Autodesk Inventor part; units mm, degrees
(part 3 of 3)
sketch "Sketch6" plane through (0, 0, 1.2) normal (0, 0, -1) x (-1, 0, 0)
  line L0 (5.715, -18.5) -> (4.445, -18.5) construction
  line L1 (4.445, -18.5) -> (4.445, -20.9) construction
  line L2 (4.445, -20.9) -> (5.715, -20.9) projected
  line L3 (5.715, -20.9) -> (5.715, -18.5) construction
  line L4 (3.175, -18.5) -> (1.905, -18.5) construction
  line L5 (1.905, -18.5) -> (1.905, -20.9) construction
  line L6 (1.905, -20.9) -> (3.175, -20.9) projected
  line L7 (3.175, -20.9) -> (3.175, -18.5) construction
  line L8 (0.635, -18.5) -> (-0.635, -18.5) construction
  line L9 (-0.635, -18.5) -> (-0.635, -20.9) construction
  line L10 (-0.635, -20.9) -> (0.635, -20.9) projected
  line L11 (0.635, -20.9) -> (0.635, -18.5) construction
  line L12 (-1.905, -18.5) -> (-3.175, -18.5) construction
  line L13 (-3.175, -18.5) -> (-3.175, -20.9) construction
  line L14 (-3.175, -20.9) -> (-1.905, -20.9) projected
  line L15 (-1.905, -20.9) -> (-1.905, -18.5) construction
  line L16 (-4.445, -18.5) -> (-5.715, -18.5) construction
  line L17 (-5.715, -18.5) -> (-5.715, -20.9) construction
  line L18 (-5.715, -20.9) -> (-4.445, -20.9) projected
  line L19 (-4.445, -20.9) -> (-4.445, -18.5) construction
  line L20 (-20.14, 20.9) -> (-21.39, 20.9) construction
  line L21 (-21.39, 20.9) -> (-21.39, 18.5) construction
  line L22 (-21.39, 18.5) -> (-20.14, 18.5) construction
  line L23 (-20.14, 18.5) -> (-20.14, 20.9) construction
  line L24 (-17.6, 20.9) -> (-18.85, 20.9) construction
  line L25 (-18.85, 20.9) -> (-18.85, 18.5) construction
  line L26 (-18.85, 18.5) -> (-17.6, 18.5) construction
  line L27 (-17.6, 18.5) -> (-17.6, 20.9) construction
  line L28 (21.39, 20.9) -> (20.14, 20.9) construction
  line L29 (20.14, 20.9) -> (20.14, 18.5) construction
  line L30 (20.14, 18.5) -> (21.39, 18.5) construction
  line L31 (21.39, 18.5) -> (21.39, 20.9) construction
  line L32 (18.85, 20.9) -> (17.6, 20.9) construction
  line L33 (17.6, 20.9) -> (17.6, 18.5) construction
  line L34 (17.6, 18.5) -> (18.85, 18.5) construction
  line L35 (18.85, 18.5) -> (18.85, 20.9) construction
  line L36 (5.715, -20.9) -> (4.445, -20.9) projected
  line L37 (4.445, -20.9) -> (4.445, -18.5) construction
  line L38 (5.715, -20.9) -> (4.445, -20.9)
  line L39 (4.445, -20.9) -> (4.445, -20.6)
  line L40 (4.445, -20.6) -> (5.715, -20.6)
  line L41 (5.715, -20.6) -> (5.715, -20.9)
  line L42 (3.175, -18.5) -> (3.175, -20.9) construction
  line L43 (1.905, -20.9) -> (1.905, -18.5) construction
  line L44 (3.175, -20.9) -> (1.905, -20.9)
  line L45 (1.905, -20.9) -> (1.905, -20.6)
  line L46 (1.905, -20.6) -> (3.175, -20.6)
  line L47 (3.175, -20.6) -> (3.175, -20.9)
  line L48 (0.635, -18.5) -> (0.635, -20.9) construction
  line L49 (-0.635, -20.9) -> (-0.635, -18.5) construction
  line L50 (0.635, -20.9) -> (-0.635, -20.9)
  line L51 (-0.635, -20.9) -> (-0.635, -20.6)
  line L52 (-0.635, -20.6) -> (0.635, -20.6)
  line L53 (0.635, -20.6) -> (0.635, -20.9)
  line L54 (-1.905, -20.9) -> (-3.175, -20.9) projected
  line L55 (-1.905, -20.9) -> (-3.175, -20.9)
  line L56 (-3.175, -20.9) -> (-3.175, -20.6)
  line L57 (-3.175, -20.6) -> (-1.905, -20.6)
  line L58 (-1.905, -20.6) -> (-1.905, -20.9)
  line L59 (-4.445, -18.5) -> (-4.445, -20.9) construction
  line L60 (-5.715, -20.9) -> (-5.715, -18.5) construction
  line L61 (-4.445, -20.9) -> (-5.715, -20.9)
  line L62 (-5.715, -20.9) -> (-5.715, -20.6)
  line L63 (-5.715, -20.6) -> (-4.445, -20.6)
  line L64 (-4.445, -20.6) -> (-4.445, -20.9)
  line L65 (20.14, 20.9) -> (21.39, 20.9) projected
  line L66 (20.14, 18.5) -> (20.14, 20.9) projected
  line L67 (21.39, 20.9) -> (20.14, 20.9)
  line L68 (20.14, 20.9) -> (20.14, 20.6)
  line L69 (20.14, 20.6) -> (21.39, 20.6)
  line L70 (21.39, 20.6) -> (21.39, 20.9)
  line L71 (17.6, 20.9) -> (18.85, 20.9) projected
  line L72 (17.6, 18.5) -> (17.6, 20.9) projected
  line L73 (18.85, 20.9) -> (17.6, 20.9)
  line L74 (17.6, 20.9) -> (17.6, 20.6)
  line L75 (17.6, 20.6) -> (18.85, 20.6)
  line L76 (18.85, 20.6) -> (18.85, 20.9)
  line L77 (-18.85, 20.9) -> (-17.6, 20.9) projected
  line L78 (-18.85, 18.5) -> (-18.85, 20.9) projected
  line L79 (-17.6, 20.9) -> (-18.85, 20.9)
  line L80 (-18.85, 20.9) -> (-18.85, 20.6)
  line L81 (-18.85, 20.6) -> (-17.6, 20.6)
  line L82 (-17.6, 20.6) -> (-17.6, 20.9)
  line L83 (-20.14, 20.9) -> (-20.14, 18.5) projected
  line L84 (-21.39, 18.5) -> (-21.39, 20.9) projected
  line L85 (-20.14, 20.9) -> (-21.39, 20.9)
  line L86 (-21.39, 20.9) -> (-21.39, 20.6)
  line L87 (-21.39, 20.6) -> (-20.14, 20.6)
  line L88 (-20.14, 20.6) -> (-20.14, 20.9)
  point P0 (0, 0)
  dimension "d37" = 0.3
  dimension "d38" = 0.3
  constraints: 72 end point, 18 parallel, 14 point on line, 9 horizontal, 9 perpendicular, 2 collinear
  measures "d37" distance between parallel lines of L2 L40
  measures "d38" distance of L68.end L67.end
extrude "Extrusion5" add sketch "Sketch6" along normal blind 2.5 bodies 4
sketch "Sketch7" plane through (0, 0, -1.3) normal (0, 0, -1) x (-1, 0, 0)
  line L0 (5.715, -20.9) -> (5.715, -20.6) construction
  line L1 (5.715, -20.6) -> (4.445, -20.6) construction
  line L2 (4.445, -20.6) -> (4.445, -20.9) construction
  line L3 (4.445, -20.9) -> (5.715, -20.9) construction
  line L4 (1.905, -20.9) -> (3.175, -20.9) construction
  line L5 (3.175, -20.9) -> (3.175, -20.6) construction
  line L6 (3.175, -20.6) -> (1.905, -20.6) construction
  line L7 (1.905, -20.6) -> (1.905, -20.9) construction
  line L8 (-0.635, -20.9) -> (0.635, -20.9) construction
  line L9 (0.635, -20.9) -> (0.635, -20.6) construction
  line L10 (0.635, -20.6) -> (-0.635, -20.6) construction
  line L11 (-0.635, -20.6) -> (-0.635, -20.9) construction
  line L12 (-1.905, -20.9) -> (-1.905, -20.6) construction
  line L13 (-1.905, -20.6) -> (-3.175, -20.6) construction
  line L14 (-3.175, -20.6) -> (-3.175, -20.9) construction
  line L15 (-3.175, -20.9) -> (-1.905, -20.9) construction
  line L16 (-5.715, -20.9) -> (-4.445, -20.9) construction
  line L17 (-4.445, -20.9) -> (-4.445, -20.6) construction
  line L18 (-4.445, -20.6) -> (-5.715, -20.6) construction
  line L19 (-5.715, -20.6) -> (-5.715, -20.9) construction
  line L20 (-20.14, 20.9) -> (-21.39, 20.9) construction
  line L21 (-21.39, 20.9) -> (-21.39, 20.6) construction
  line L22 (-21.39, 20.6) -> (-20.14, 20.6) construction
  line L23 (-20.14, 20.6) -> (-20.14, 20.9) construction
  line L24 (-17.6, 20.9) -> (-18.85, 20.9) construction
  line L25 (-18.85, 20.9) -> (-18.85, 20.6) construction
  line L26 (-18.85, 20.6) -> (-17.6, 20.6) construction
  line L27 (-17.6, 20.6) -> (-17.6, 20.9) construction
  line L28 (21.39, 20.9) -> (20.14, 20.9) construction
  line L29 (20.14, 20.9) -> (20.14, 20.6) construction
  line L30 (20.14, 20.6) -> (21.39, 20.6) construction
  line L31 (21.39, 20.6) -> (21.39, 20.9) construction
  line L32 (18.85, 20.9) -> (17.6, 20.9) construction
  line L33 (17.6, 20.9) -> (17.6, 20.6) construction
  line L34 (17.6, 20.6) -> (18.85, 20.6) construction
  line L35 (18.85, 20.6) -> (18.85, 20.9) construction
  line L36 (5.715, -20.9) -> (4.445, -20.9) projected
  line L37 (4.445, -20.6) -> (5.715, -20.6) projected
  line L38 (5.33, -20.9) -> (4.83, -20.9)
  line L39 (4.83, -20.9) -> (4.83, -20.6)
  line L40 (4.83, -20.6) -> (5.33, -20.6)
  line L41 (5.33, -20.6) -> (5.33, -20.9)
  line L42 (3.175, -20.9) -> (1.905, -20.9) projected
  line L43 (2.79, -20.9) -> (2.29, -20.9)
  line L44 (2.29, -20.9) -> (2.29, -20.6)
  line L45 (2.29, -20.6) -> (2.79, -20.6)
  line L46 (2.79, -20.6) -> (2.79, -20.9)
  line L47 (0.635, -20.9) -> (-0.635, -20.9) projected
  line L48 (0.25, -20.9) -> (-0.25, -20.9)
  line L49 (-0.25, -20.9) -> (-0.25, -20.6)
  line L50 (-0.25, -20.6) -> (0.25, -20.6)
  line L51 (0.25, -20.6) -> (0.25, -20.9)
  line L52 (-1.905, -20.9) -> (-3.175, -20.9) projected
  line L53 (-3.175, -20.6) -> (-1.905, -20.6) projected
  line L54 (-2.29, -20.9) -> (-2.79, -20.9)
  line L55 (-2.79, -20.9) -> (-2.79, -20.6)
  line L56 (-2.79, -20.6) -> (-2.29, -20.6)
  line L57 (-2.29, -20.6) -> (-2.29, -20.9)
  line L58 (-4.445, -20.9) -> (-5.715, -20.9) projected
  line L59 (-5.715, -20.6) -> (-4.445, -20.6) projected
  line L60 (-4.83, -20.9) -> (-5.33, -20.9)
  line L61 (-5.33, -20.9) -> (-5.33, -20.6)
  line L62 (-5.33, -20.6) -> (-4.83, -20.6)
  line L63 (-4.83, -20.6) -> (-4.83, -20.9)
  line L64 (20.14, 20.9) -> (21.39, 20.9) projected
  line L65 (21.39, 20.6) -> (20.14, 20.6) projected
  line L66 (21.015, 20.9) -> (20.515, 20.9)
  line L67 (20.515, 20.9) -> (20.515, 20.6)
  line L68 (20.515, 20.6) -> (21.015, 20.6)
  line L69 (21.015, 20.6) -> (21.015, 20.9)
  line L70 (17.6, 20.9) -> (18.85, 20.9) projected
  line L71 (18.85, 20.6) -> (17.6, 20.6) projected
  line L72 (18.475, 20.9) -> (17.975, 20.9)
  line L73 (17.975, 20.9) -> (17.975, 20.6)
  line L74 (17.975, 20.6) -> (18.475, 20.6)
  line L75 (18.475, 20.6) -> (18.475, 20.9)
  line L76 (-18.85, 20.9) -> (-17.6, 20.9) projected
  line L77 (-17.6, 20.6) -> (-18.85, 20.6) projected
  line L78 (-17.975, 20.9) -> (-18.475, 20.9)
  line L79 (-18.475, 20.9) -> (-18.475, 20.6)
  line L80 (-18.475, 20.6) -> (-17.975, 20.6)
  line L81 (-17.975, 20.6) -> (-17.975, 20.9)
  line L82 (-21.39, 20.9) -> (-20.14, 20.9) projected
  line L83 (-20.14, 20.6) -> (-21.39, 20.6) projected
  line L84 (-20.515, 20.9) -> (-21.015, 20.9)
  line L85 (-21.015, 20.9) -> (-21.015, 20.6)
  line L86 (-21.015, 20.6) -> (-20.515, 20.6)
  line L87 (-20.515, 20.6) -> (-20.515, 20.9)
  point P0 (0, 0)
  point P1 (5.08, -20.9)
  point P2 (5.08, -20.9)
  point P3 (2.54, -20.9)
  point P4 (2.54, -20.9)
  point P5 (0, -20.9)
  point P6 (0, -20.9)
  point P7 (-2.54, -20.9)
  point P8 (-2.54, -20.9)
  point P9 (-5.08, -20.9)
  point P10 (-5.08, -20.9)
  point P11 (-18.225, 20.6)
  point P12 (-18.225, 20.6)
  point P13 (-20.765, 20.6)
  point P14 (-20.765, 20.6)
  point P15 (18.225, 20.6)
  point P16 (18.225, 20.6)
  point P17 (20.765, 20.6)
  point P18 (20.765, 20.6)
  dimension "d41" = 0.5
  dimension "d42" = 0.5
  dimension "d43" = 0.5
  dimension "d44" = 0.5
  dimension "d45" = 0.5
  dimension "d46" = 0.5
  dimension "d47" = 0.5
  dimension "d48" = 0.5
  dimension "d49" = 0.5
  constraints: 72 end point, 18 midpoint, 18 parallel, 18 point on line, 9 coincident, 9 horizontal, 9 perpendicular
  measures "d41" distance between parallel lines of L39 L41
  measures "d42" distance between parallel lines of L44 L46
  measures "d43" distance between parallel lines of L49 L51
  measures "d44" distance between parallel lines of L55 L57
  measures "d45" distance between parallel lines of L61 L63
  measures "d46" distance between parallel lines of L67 L69
  measures "d47" distance between parallel lines of L73 L75
  measures "d48" distance between parallel lines of L79 L81
  measures "d49" distance between parallel lines of L85 L87
extrude "Extrusion6" add sketch "Sketch7" along normal blind 3.4 bodies 4
sketch "Sketch8" plane through (0, 0, 0) normal (0, 0, -1) x (-1, 0, 0)
  arc A0 (24.7705, 6.35) -> (23.765, 7.25) centre (23.865, 6.35) ccw projected
  line L0 (23.765, 20.5) -> (23.765, 7.25) projected
  line L1 (-23.765, 20.5) -> (23.765, 20.5) projected
  line L2 (-23.765, -20.5) -> (-23.765, 20.5) projected
  line L3 (23.765, -20.5) -> (-23.765, -20.5) projected
  line L4 (23.765, -2.75) -> (23.765, -20.5) projected
  arc A1 (23.765, -2.75) -> (24.7705, -1.85) centre (23.865, -1.85) ccw projected
  line L5 (24.7705, 6.35) -> (24.7705, -1.85) projected
  line L6 (-24, 20) -> (24, 20)
  line L7 (24, 20) -> (24, -20)
  line L8 (24, -20) -> (-24, -20)
  line L9 (-24, -20) -> (-24, 20)
  point P0 (0, 0)
  point P1 (-24, 0)
  point P2 (-23.765, 0)
  point P3 (0, 20)
  dimension "d52" = 48
  dimension "d53" = 40
  constraints: 8 end point, 3 midpoint, 2 parallel, 1 horizontal, 1 horizontal alignment, 1 perpendicular, 1 vertical alignment
  measures "d52" distance between parallel lines of L7 L9
  measures "d53" distance between parallel lines of L8 L6
extrude "Extrusion7" [suppressed]
sketch "Sketch9" plane through (0, 0, 1.2) normal (0, 0, 1) x (1, 0, 0)
  arc A0 (-23.765, 7.25) -> (-24.7705, 6.35) centre (-23.865, 6.35) ccw
  line L0 (-24.7705, 6.35) -> (-24.7705, -1.85)
  arc A1 (-24.7705, -1.85) -> (-23.765, -2.75) centre (-23.865, -1.85) ccw
  line L1 (-23.765, -2.75) -> (-23.765, -20.5)
  line L2 (-23.765, -20.5) -> (23.765, -20.5)
  line L3 (23.765, -20.5) -> (23.765, 20.5)
  line L4 (23.765, 20.5) -> (-23.765, 20.5)
  line L5 (-23.765, 20.5) -> (-23.765, 7.25)
  arc A2 (-23.765, 7.25) -> (-24.7705, 6.35) centre (-23.865, 6.35) ccw
  line L6 (-24.7705, 6.35) -> (-24.7705, -1.85)
  arc A3 (-24.7705, -1.85) -> (-23.765, -2.75) centre (-23.865, -1.85) ccw
  line L7 (-23.765, -2.75) -> (-23.765, -14)
  line L8 (-23.765, -14) -> (23.765, -14)
  line L9 (23.765, -14) -> (23.765, 18.5)
  line L10 (23.765, 18.5) -> (-23.765, 18.5)
  line L11 (-23.765, 18.5) -> (-23.765, 7.25)
  line L12 (-4.445, -18.5) -> (-5.715, -18.5)
  line L13 (-5.715, -18.5) -> (-5.715, -20.9)
  line L14 (-5.715, -20.9) -> (-4.445, -20.9)
  line L15 (-4.445, -20.9) -> (-4.445, -18.5)
  line L16 (-1.905, -18.5) -> (-3.175, -18.5)
  line L17 (-3.175, -18.5) -> (-3.175, -20.9)
  line L18 (-3.175, -20.9) -> (-1.905, -20.9)
  line L19 (-1.905, -20.9) -> (-1.905, -18.5)
  line L20 (0.635, -18.5) -> (-0.635, -18.5)
  line L21 (-0.635, -18.5) -> (-0.635, -20.9)
  line L22 (-0.635, -20.9) -> (0.635, -20.9)
  line L23 (0.635, -20.9) -> (0.635, -18.5)
  line L24 (3.175, -18.5) -> (1.905, -18.5)
  line L25 (1.905, -18.5) -> (1.905, -20.9)
  line L26 (1.905, -20.9) -> (3.175, -20.9)
  line L27 (3.175, -20.9) -> (3.175, -18.5)
  line L28 (5.715, -18.5) -> (4.445, -18.5)
  line L29 (4.445, -18.5) -> (4.445, -20.9)
  line L30 (4.445, -20.9) -> (5.715, -20.9)
  line L31 (5.715, -20.9) -> (5.715, -18.5)
  line L32 (-23.765, -20.5) -> (23.765, -20.5)
  line L33 (-23.765, -14) -> (23.765, -14)
  line L34 (23.765, -14) -> (23.765, -20.5)
  line L35 (23.765, -20.5) -> (-23.765, -20.5)
  line L36 (-23.765, -20.5) -> (-23.765, -14)
extrude "Extrusion8" add sketch "Sketch9" along normal blind 0.15 separate body contours L3 L2 L31 L28 L29 L27 L24 L25 L23 L20 L21 L19 L16 L17 L15 L12 L13 L1 L8 | L2 L29 L28 L31 | L13 L12 L15 L2 | L2 L25 L24 L27 | L17 L16 L19 L2 | L2 L21 L20 L23
body "Solid1"
body "Solid2"
body "Solid3"
body "Solid4"
body "Solid5"
body "Solid6"
